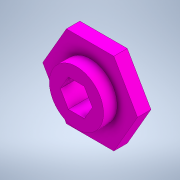
# Autodesk Inventor part: 1_2x1-hexBushing
Saved by Autodesk Inventor 2021.2 (Build 252289000, 289)
## iProperties
Created: 2020-11-08
Part Number: 1_2x1-hexBushing
Material: PC/ABS Plastic
Document SubType Name: Modeling
Designer: robst
Density: 0.357273 g/cm^3
Appearance: Magenta
Author: robst
Autodesk Inventor part; units mm, degrees
ref_plane "YZ Plane" through (0, 0, 0) normal (1, 0, 0) x (0, 1, 0)
ref_plane "XZ Plane" through (0, 0, 0) normal (0, 1, 0) x (-1, 0, 0)
ref_plane "XY Plane" through (0, 0, 0) normal (0, 0, 1) x (1, 0, 0)
sketch "Sketch1" plane through (0, 0, 0) normal (0, 0, 1) x (1, 0, 0)
  line L0 (3.6662, 6.35) -> (7.3323, 0)
  line L1 (7.3323, 0) -> (3.6662, -6.35)
  line L2 (3.6662, -6.35) -> (-3.6662, -6.35)
  line L3 (-3.6662, -6.35) -> (-7.3323, 0)
  line L4 (-7.3323, 0) -> (-3.6662, 6.35)
  line L5 (-3.6662, 6.35) -> (3.6662, 6.35)
  circle A0 centre (0, 0) radius 12.7
  circle A1 centre (0, 0) radius 7.3323 construction
  dimension "d0" = 12.7
  dimension "d2" = 25.4
  dimension "d3" = 5.3677
  constraints: 12 end point, 3 coincident, 1 centre point, 1 horizontal, 1 horizontal alignment, 15 other
  measures "d0" distance between parallel lines of L2 L5
  measures "d2" diameter of A0
extrude "Extrusion1" add sketch "Sketch1" against normal blind 6.35
sketch "Sketch2" plane through (0, 0, -6.35) normal (0, 0, -1) x (-1, 0, 0)
  line L0 (7.3323, 0) -> (3.6662, -6.35) projected
  line L1 (3.6662, -6.35) -> (-3.6662, -6.35)
  line L2 (-3.6662, -6.35) -> (-7.3323, 0)
  line L3 (-7.3323, 0) -> (-3.6662, 6.35)
  line L4 (-3.6662, 6.35) -> (3.6662, 6.35)
  line L5 (3.6662, 6.35) -> (7.3323, 0)
  line L6 (7.3323, 0) -> (3.6662, -6.35)
  line L7 (-10.9985, 19.05) -> (10.9985, 19.05)
  line L8 (10.9985, 19.05) -> (21.997, 0)
  line L9 (21.997, 0) -> (10.9985, -19.05)
  line L10 (10.9985, -19.05) -> (-10.9985, -19.05)
  line L11 (-10.9985, -19.05) -> (-21.997, 0)
  line L12 (-21.997, 0) -> (-10.9985, 19.05)
  point P0 (0, 0)
  point P1 (0, 0)
  point P2 (0, 0)
  dimension "d7" = 12.7
  dimension "d10" = 38.1
  constraints: 24 end point, 1 coincident, 1 collinear, 1 horizontal, 26 other
  measures "d7" distance between parallel lines of L3 L6
  measures "d10" distance between parallel lines of L10 L7
extrude "Extrusion3" add sketch "Sketch2" along normal blind 6.35
thicken "Thicken Internal Hex Hold" operation add thickness 0.127 both sides no extend neighbours yes toward (0, 1, 0) faces at (1.2221, 6.35, -8.4667) (-4.8882, 4.2333, -8.4667) (1.2221, 14.8167, -12.7) (6.1103, -2.1167, -8.4667) (1.2221, -6.35, -8.4667) (-4.8882, -4.2333, -4.2333)
thicken "Reduce Size of Bushing Fitting" operation add thickness 0.127 both sides no extend neighbours yes toward (-0.9967573, 0.0804666, 0) faces at (12.6588, -1.0219, -4.2333)
equation "\"d13\" = printSpacing"
equation "\"d14\" = printSpacing"
equation "\"d15\" = printSpacing"
equation "\"d16\" = printSpacing"
equation "\"hexSize\" = 12.7"
equation "\"printSpacing\" = 0.127"
body "Solid1"
